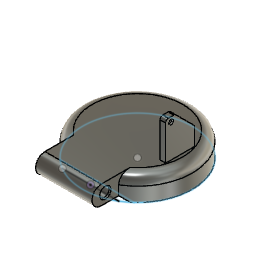
Cookie jar lidt v2 (Autodesk Fusion 360 design; units mm, degrees)
Autodesk Fusion 360 part; units mm, degrees
sketch "Sketch1" plane through (0, 0, 0) normal (0, 0, 1) x (1, 0, 0)
  line L0 (0, 0) -> (30, 0)
  line L1 (0, 0) -> (-30, 0)
  circle A0 centre (0, 50) radius 58.3095
  line L2 (0, 7) -> (39.3827, 7)
  line L3 (0, 7) -> (-39.3827, 7)
  dimension "d1" = 30
  dimension "d2" = 7
  constraint coincident L0.start L1.start
  constraint horizontal L0
  constraint parallel L0 L1
  constraint coincident L0.end A0
  constraint coincident A0 L2.end
  constraint coincident A0 L3.end
  measures "d1" distance of L0.start L0.end
  measures "d2" distance of L0.start L2.start
extrude "Extrude1" add sketch "Sketch1" along normal blind 25 contours A0 L2 L3
extrude "Extrude2" add sketch "Sketch1" along normal blind 25 contours L0 L1 A0 L2 L3
sketch "Sketch2" plane through (0, 0, 0) normal (0, -1, 0) x (1, 0, 0)
  line L0 (-30, 0) -> (30, 0)
  line L1 (30, 0) -> (30, 25)
  line L2 (30, 25) -> (-30, 25)
  line L3 (-30, 25) -> (-30, 0)
  line L4 (-30, 0) -> (-30, 10)
  line L5 (30, 0) -> (30, 5)
  line L6 (30, 5) -> (-30, 5)
  dimension "d7" = 10
  dimension "d8" = 5
  constraint coincident L0.start L3.end
  constraint perpendicular L0 L4
  constraint coincident L0.end L1.start
  constraint perpendicular L0 L5
  constraint midpoint L4 L6.end
  measures "d7" distance of L0.start L4.end
  measures "d8" distance of L0.end L5.end
chamfer "Chamfer1" distance 5 angle 45 1 edges at (0, 0, 0)
extrude "Extrude3" add sketch "Sketch2" along normal blind 28.5 contours L1 L2 L3 L4 L6
sketch "Sketch3" plane through (-30, 0, 0) normal (-1, 0, 0) x (0, -1, 0)
  line L0 (0, 25) -> (0, 5)
  line L1 (0, 5) -> (28.5, 5)
  line L2 (28.5, 5) -> (28.5, 25)
  line L3 (28.5, 25) -> (0, 25)
  line L4 (28.5, 25) -> (14.25, 25)
  line L5 (14.25, 25) -> (14.25, 15)
  circle A0 centre (14.25, 15) radius 5
  dimension "d12" = 10
  dimension "d13" = 10
  constraint coincident L2.end L3.start
  constraint midpoint L3 L4.end
  constraint perpendicular L4 L5
  constraint coincident L5.end A0.centre
  measures "d12" distance of L4.end L5.end
  measures "d13" diameter of A0
extrude "Extrude4" cut sketch "Sketch3" against normal blind 60 contours A0
fillet "Fillet1" radius 1 2 edges at (-30, -9.5884, 16.8081) (30, -9.5884, 13.1919)
fillet "Fillet2" radius 10 2 edges at (0, -28.5, 25) (0, -28.5, 5)
fillet "Fillet3" radius 10 1 edges at (0, 108.3095, 25)
sketch "Sketch4" plane through (0, 0, 25) normal (0, 0, 1) x (-1, 0, 0)
  line L0 (30, -12.1343) -> (30, 18.5)
  line L1 (30, 18.5) -> (-30, 18.5)
  line L2 (-30, 18.5) -> (-30, -12.1343)
  arc A0 (-30, -12.1343) -> (30, -12.1343) centre (0, -50) ccw
  line L3 (-30, -12.1343) -> (-30, -35)
  line L4 (-30, -35) -> (-42, -35)
  line L5 (-42, -35) -> (-45, -35)
  line L6 (-45, -35) -> (-39, -35)
  line L7 (-39, -35) -> (-39, -66)
  line L8 (-39, -66) -> (-45, -66)
  line L9 (-45, -66) -> (-45, -35)
  dimension "d22" = 12
  dimension "d23" = 3
  constraint coincident L2.end A0.start
  constraint parallel L2 L3
  constraint perpendicular L3 L4
  constraint parallel L4 L5
  constraint horizontal L6
  constraint vertical L7
  constraint horizontal L8
  constraint vertical L9
  measures "d22" distance of L3.end L4.end
  measures "d23" distance of L4.end L5.end
extrude "Extrude5" add sketch "Sketch4" along normal blind 40 contours L4 L5 L6 L7 L8 L9
chamfer "Chamfer2" distance 21 angle 45 1 edges at (42, 66, 65)
fillet "Fillet4" radius 3 3 edges at (42, 35, 65) (42, 45, 65) (42, 66, 44)
sketch "Sketch5" plane through (45, 0, 0) normal (1, 0, 0) x (0, 1, 0)
  arc A0 (66, 42.7574) -> (65.1213, 44.8787) centre (63, 42.7574) ccw
  line L0 (65.1213, 44.8787) -> (45.8787, 64.1213)
  arc A1 (45.8787, 64.1213) -> (43.7574, 65) centre (43.7574, 62) ccw
  line L1 (43.7574, 65) -> (38, 65)
  arc A2 (38, 65) -> (35, 62) centre (38, 62) ccw
  line L2 (35, 62) -> (35, 25)
  line L3 (35, 25) -> (66, 25)
  line L4 (66, 25) -> (66, 42.7574)
  circle A3 centre (40.8787, 60) radius 1.5
  dimension "d29" = 3
  measures "d29" diameter of A3
extrude "Extrude6" cut sketch "Sketch5" against normal blind 6 contours A3
fillet "Fillet5" radius 1 2 edges at (39, 39.4802, 59.4576) (45, 39.4802, 60.5424)
